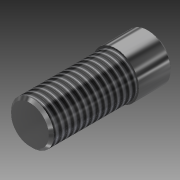
# Autodesk Inventor part: BUSS-STUD-250X50
Saved by Autodesk Inventor 2013 (Build 170138000, 138)
## iProperties
Shininess: 64.0
Length Units: 11272
Angle Units: 11279
Time Units: 11290
Mass Units: 11286
Length Display Precision: 3
Angle Display Precision: 2
Compacted: True
Part Number: BUSS-STUD-250X50
Document SubType Name: Modeling
Created: 2003-01-12
Designer: geyerm
Material: Steel, High Strength Low Alloy
Density: 7.84 g/cm^3
Density: 0.0
Volumn: 0.0
Area: 0.0
PropertySet Name: Model Information
Control State: 0
Master: False
Checked Out: False
Author: Autodesk
Autodesk Inventor part; units mm, degrees
ref_plane "YZ Plane" through (0, 0, 0) normal (1, 0, 0) x (0, 1, 0)
ref_plane "XZ Plane" through (0, 0, 0) normal (0, 1, 0) x (-1, 0, 0)
ref_plane "XY Plane" through (0, 0, 0) normal (0, 0, 1) x (1, 0, 0)
sketch "Sketch1" plane through (0, 0, 0) normal (0, 0, 1) x (1, 0, 0)
  circle A0 centre (-34.8653, 6.0523) radius 3.429 projected
  circle A1 centre (-34.8653, 6.0523) radius 3.429
  dimension "d0" = 6.858
  constraints: 1 centre point, 1 coincident, 1 concentric
  measures "d0" diameter of A1
extrude "Extrusion1" add sketch "Sketch1" against normal blind 5.08
chamfer "Chamfer1" distance 0.381 angle 45 1 edges at (-38.2943, 6.0523, -5.08)
sketch "Sketch2" plane through (-34.8653, 6.0523, 0) normal (0, 0, 1) x (1, 0, 0)
  circle A0 centre (0, 0) radius 3.429 projected
  circle A1 centre (0, 0) radius 3.175
  dimension "d5" = 6.35
  constraints: 1 centre point, 1 coincident, 1 concentric
  measures "d5" diameter of A1
extrude "Extrusion2" add sketch "Sketch2" along normal blind 12.7 contours A1
chamfer "Chamfer2" distance 0.381 angle 45 1 edges at (-38.0403, 6.0523, 12.7)
thread "Thread1" size "1/4-28 UNF" class "1A" standard "ANSI Unified Screw Threads" full length
body "Solid1"
